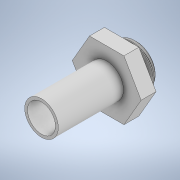
# Autodesk Inventor part: WaterAdapter
Saved by Autodesk Inventor 2021 (Build 250183000, 183)
## iProperties
Created: 2021-01-28
Part Number: WaterAdapter
Material: Generic
Document SubType Name: Modeling
Designer: Timo
Density: 1 g/cm^3
Appearance: Default
Author: Timo
Autodesk Inventor part; units mm, degrees
ref_plane "YZ Plane" through (0, 0, 0) normal (1, 0, 0) x (0, 1, 0)
ref_plane "XZ Plane" through (0, 0, 0) normal (0, 1, 0) x (-1, 0, 0)
ref_plane "XY Plane" through (0, 0, 0) normal (0, 0, 1) x (1, 0, 0)
sketch "Sketch1" plane through (0, 0, 0) normal (0, 0, 1) x (1, 0, 0)
  line L0 (-9.2376, 16) -> (9.2376, 16)
  line L1 (9.2376, 16) -> (18.4752, 0)
  line L2 (18.4752, 0) -> (9.2376, -16)
  line L3 (9.2376, -16) -> (-9.2376, -16)
  line L4 (-9.2376, -16) -> (-18.4752, 0)
  line L5 (-18.4752, 0) -> (-9.2376, 16)
  point P0 (0, 0)
  point P1 (0, 0)
  dimension "d0" = 32
  constraints: 12 end point, 1 coincident, 1 horizontal, 13 other
  measures "d0" distance between parallel lines of L3 L0
extrude "Extrusion1" add sketch "Sketch1" along normal blind 8
sketch "Sketch2" plane through (0, 0, 0) normal (0, 0, -1) x (-1, 0, 0)
  circle A0 centre (0, 0) radius 9.925
  dimension "d3" = 19.85
  constraints: 1 centre point, 1 coincident
  measures "d3" diameter of A0
extrude "Extrusion2" add sketch "Sketch2" along normal blind 8
sketch "Sketch3" plane through (0, 0, 0) normal (1, 0, 0) x (0, 1, 0)
  line L0 (9.925, 2.6258) -> (12.199, 1.3129)
  line L1 (12.199, 1.3129) -> (9.925, 0)
  line L2 (9.925, 0) -> (9.925, 2.6258)
  line L3 (11.75, 11.6995) -> (11.75, -11.0204) construction
  line L4 (10.9, -10.7686) -> (10.9, 10.1882) construction
  line L5 (9.925, 10.9583) -> (9.925, -10.6881) construction
  line L6 (16, 0) -> (0, 0) construction
  line L7 (11.75, 1.0537) -> (11.75, 1.5722)
  point P0 (10.9, 2.0629)
  point P1 (10.9, 0.5629)
  dimension "d6" = 19.85
  dimension "d7" = 21.8
  dimension "d8" = 23.5
  dimension "d9" = 30
  dimension "d10" = 60
  dimension "d11" = 1.5
  constraints: 14 end point, 11 point on line, 3 vertical
  measures "d6" diameter of L6.end L5
  measures "d7" diameter of L6.end L4
  measures "d8" diameter of L6.end L3
  measures "d9" angle of L6 L1
  measures "d10" angle of L1 L0
  measures "d11" distance of point (10.9, 2.063) point (10.9, 0.563)
coil "Coil1" sketch "Sketch3" operation add axis through (0, 0, -10) along (0, 0, -1) pitch 3 turns 5 hand right contours L0 L7 L1 L2
sketch "Sketch4" plane through (0, 0, -8) normal (0, 0, -1) x (-1, 0, 0)
  circle A0 centre (0, 0) radius 16.7379
  constraints: 1 centre point, 1 coincident
extrude "Extrusion3" cut sketch "Sketch4" along normal blind 8
sketch "Sketch5" plane through (0, 0, 0) normal (1, 0, 0) x (0, 1, 0)
  line L0 (11.8, -6.2) -> (10, -8)
  line L1 (10, -8) -> (11.8, -8)
  line L2 (11.8, -8) -> (11.8, -6.2)
  line L3 (11.6759, -8) -> (-4.9625, -8) projected
  line L4 (0, -9.6) -> (0, 1.6) projected
  point P0 (0, 0)
  dimension "d22" = 10
  dimension "d23" = 11.8
  dimension "d24" = 45
  constraints: 6 end point, 1 horizontal, 1 perpendicular, 1 point on line
  measures "d22" horizontal distance of point (0, 0) L0.end
  measures "d23" horizontal distance of point (0, 0) L1.end
  measures "d24" angle of L0 L1
revolve "Revolution1" cut sketch "Sketch5" angle 360 about axis through (0, 0, -10) along (0, 0, 1)
sketch "Sketch6" plane through (0, 0, 8) normal (0, 0, 1) x (1, 0, 0)
  circle A0 centre (0, 0) radius 9
  dimension "d26" = 18
  constraints: 1 centre point, 1 coincident
  measures "d26" diameter of A0
extrude "Extrusion4" add sketch "Sketch6" along normal blind 35
sketch "Sketch7" plane through (0, 0, 43) normal (0, 0, 1) x (1, 0, 0)
  circle A0 centre (0, 0) radius 9 projected
  circle A1 centre (0, 0) radius 7.5
  dimension "d29" = 1.5
  constraints: 1 centre point
  measures "d29" radial gap between concentric circles of A0 A1
extrude "Extrusion5" cut sketch "Sketch7" against normal through all contours A1
body "Solid1"
